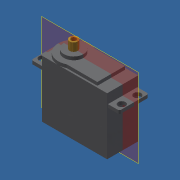
# Autodesk Inventor part: servo
Saved by Autodesk Inventor 2016 (Build 200138000, 138)
## iProperties
Created: 2013-01-25
Part Number: servo
Document SubType Name: Modeling
Designer: jörg
Density: 1.493 g/cm^3
Material: PC/ABS-Kunststoff
Mass: 42.3132 g
Surface Area: 66.0322 cm^2
Volume: 28.341 cm^3
Appearance: Glatt - mittelgrau
Author: jörg
Autodesk Inventor part; units mm, degrees
ref_plane "YZ Plane" through (0, 0, 0) normal (1, 0, 0) x (0, 1, 0)
ref_plane "XZ Plane" through (0, 0, 0) normal (0, 1, 0) x (-1, 0, 0)
ref_plane "XY Plane" through (0, 0, 0) normal (0, 0, 1) x (1, 0, 0)
sketch "Skizze1" plane through (0, 0, 0) normal (0, 0, 1) x (1, 0, 0)
  line L0 (0, 0) -> (-40, 0)
  line L1 (-40, 0) -> (-40, 19)
  line L2 (-40, 19) -> (0, 19)
  line L3 (0, 19) -> (0, 0)
  dimension "d0" = 40
  dimension "d1" = 19
  constraints: 8 end point, 2 parallel, 1 horizontal, 1 perpendicular
  measures "d0" distance of L1.end L2.end
  measures "d1" distance of L0.end L1.end
extrude "Extrusion1" add sketch "Skizze1" along normal blind 35
sketch "Skizze2" plane through (0, 0, 35) normal (0, 0, 1) x (1, 0, 0)
  line L0 (-40, 19) -> (0, 19) projected
  circle A0 centre (-30, 9.5) radius 9.5
  dimension "d4" = 10
  constraints: 1 centre point, 1 tangent
  measures "d4" horizontal distance of L0.start A0.centre
extrude "Extrusion2" add sketch "Skizze2" along normal blind 2
sketch "Skizze3" plane through (0, 0, 35) normal (0, 0, 1) x (1, 0, 0)
  line L0 (0, 19) -> (0, 0) projected
  line L1 (-37, 3.6605) -> (-37, 17.3389)
  line L2 (-7, 1) -> (-7, 18)
  line L3 (-7, 18) -> (-30, 18)
  line L4 (-30, 18) -> (-30, 1)
  line L5 (-30, 1) -> (-7, 1)
  dimension "d13" = 17
  constraints: 10 end point, 3 parallel, 1 perpendicular
  measures "d13" distance of L2.start L2.end
extrude "Extrusion3" add sketch "Skizze3" along normal blind 2
sketch "Skizze4" plane through (0, 0, 37) normal (0, 0, 1) x (1, 0, 0)
  arc A0 (-25.7574, 18) -> (-25.7574, 1) centre (-30, 9.5) ccw projected
  circle A1 centre (-30, 9.5) radius 6
  point P0 (0, 0)
  dimension "d16" = 12
  constraints: 1 centre point, 1 coincident
  measures "d16" diameter of A1
extrude "Extrusion4" add sketch "Skizze4" along normal blind 2
sketch "Skizze6" plane through (-40, 0, 0) normal (-1, 0, 0) x (0, 0, 1)
  line L0 (27, 18.5) -> (29, 18.5)
  line L1 (29, 18.5) -> (29, 0.5)
  line L2 (29, 0.5) -> (27, 0.5)
  line L3 (27, 0.5) -> (27, 18.5)
  dimension "d23" = 2
  dimension "d24" = 18
  constraints: 8 end point, 2 parallel, 1 horizontal, 1 perpendicular
  measures "d23" distance of L1.end L2.end
  measures "d24" distance of L0.end L1.end
extrude "Extrusion5" add sketch "Skizze6" along normal blind 7
sketch "Skizze7" plane through (-40, 0.5, 29) normal (0, 0, 1) x (1, 0, 0)
  circle A0 centre (-4.25, 4.25) radius 2.25
  circle A1 centre (-4.25, 13.75) radius 2.25
  point P0 (40, -0.5)
  dimension "d27" = 4.5
  dimension "d28" = 4.5
  constraints: 2 centre point
  measures "d27" diameter of A0
  measures "d28" diameter of A1
extrude "Extrusion6" cut sketch "Skizze7" against normal blind 2 contours A0
sketch "Skizze8" plane through (-40, 0.5, 29) normal (0, 0, 1) x (1, 0, 0)
  circle A0 centre (-4.25, 13.75) radius 2.25
  point P0 (40, -0.5)
  dimension "d31" = 4.5
  constraints: 1 centre point
  measures "d31" diameter of A0
extrude "Extrusion7" cut sketch "Skizze8" against normal blind 2
fillet "Rundung1" radius 1 1 edges at (-47, 0.5, 28)
fillet "Rundung2" radius 1 1 edges at (-47, 18.5, 28)
sketch "Skizze9" plane through (0, 0, 0) normal (1, 0, 0) x (0, 0, -1)
  line L0 (-27, 0.5) -> (-29, 0.5)
  line L1 (-29, 0.5) -> (-29, 18.5)
  line L2 (-29, 18.5) -> (-27, 18.5)
  line L3 (-27, 18.5) -> (-27, 0.5)
  dimension "d36" = 2
  dimension "d37" = 18
  constraints: 8 end point, 2 parallel, 1 horizontal, 1 perpendicular
  measures "d36" distance of L1.end L2.end
  measures "d37" distance of L0.end L1.end
extrude "Extrusion8" add sketch "Skizze9" along normal blind 7
sketch "Skizze10" plane through (0, 0.5, 29) normal (0, 0, 1) x (1, 0, 0)
  circle A0 centre (4.25, 4.25) radius 2.25
  point P0 (0, -0.5)
  dimension "d40" = 4.5
  constraints: 1 centre point
  measures "d40" diameter of A0
extrude "Extrusion9" cut sketch "Skizze10" against normal blind 2
sketch "Skizze11" plane through (0, 0.5, 29) normal (0, 0, 1) x (1, 0, 0)
  circle A0 centre (4.25, 13.75) radius 2.25
  point P0 (0, -0.5)
  dimension "d43" = 4.5
  constraints: 1 centre point
  measures "d43" diameter of A0
extrude "Extrusion10" cut sketch "Skizze11" against normal blind 2
fillet "Rundung3" radius 1 1 edges at (7, 18.5, 28)
fillet "Rundung4" radius 1 1 edges at (7, 0.5, 28)
sketch "Skizze12" plane through (-30, 9.5, 39) normal (0, 0, 1) x (1, 0, 0)
  circle A0 centre (0, 0) radius 6 projected
  circle A1 centre (0, 0) radius 1.5
  circle A2 centre (0, 0) radius 2.5
  point P0 (30, -9.5)
  dimension "d48" = 3
  dimension "d49" = 5
  constraints: 2 centre point, 2 coincident
  measures "d48" diameter of A1
  measures "d49" diameter of A2
extrude "Extrusion11" add sketch "Skizze12" along normal blind 5 separate body contours A2
ref_plane "Arbeitsebene1" through (-40, 9.5, 0) normal (0, 1, 0) x (1, 0, 0)
